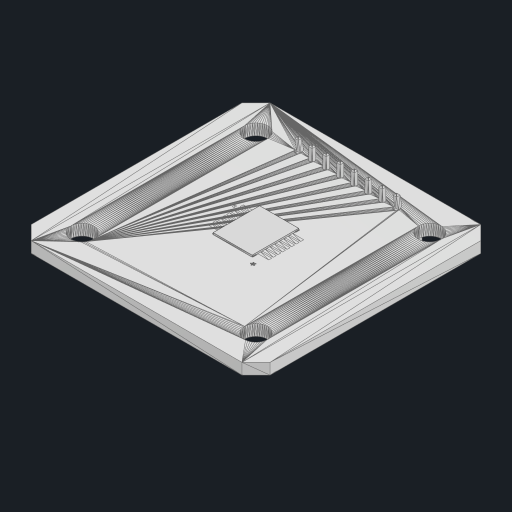
# Autodesk Inventor part: ArmEncoderBoard2
Saved by Autodesk Inventor 2023 (Build 270158000, 158)
## iProperties
Created: 2024-03-09
Part Number: ArmEncoderBoard2
Material: Generic
Document SubType Name: Modeling
Designer: valer
Density: 1 g/cm^3
Appearance: Default
Author: valer
Autodesk Inventor part; units mm, degrees
ref_plane "YZ Plane" through (0, 0, 0) normal (1, 0, 0) x (0, 1, 0)
ref_plane "XZ Plane" through (0, 0, 0) normal (0, 1, 0) x (-1, 0, 0)
ref_plane "XY Plane" through (0, 0, 0) normal (0, 0, 1) x (1, 0, 0)
ref_plane "Work Plane1" through (-14.5282, -0.6229, 20.934) normal (-0.0000001, 1, 0.0000001) x (-1, -0.0000001, 0)
sketch "Sketch1" plane through (-14.5282, -0.6229, 20.934) normal (-0.0000001, 1, 0.0000001) x (-1, -0.0000001, 0)
  line L0 (-12.2033, -20.3154) -> (-17.7585, -20.3154)
  line L1 (-17.7585, -20.3154) -> (-17.7585, -13.6964)
  line L2 (-17.7585, -13.6964) -> (-12.2033, -13.6964)
  line L3 (-12.2033, -13.6964) -> (-12.2033, -20.3154)
  point P0 (-14.5282, -20.934)
  constraints: 8 end point, 2 parallel, 1 horizontal, 1 perpendicular
extrude "Extrusion1" add sketch "Sketch1" along normal blind 0.25
body "Solid1"
